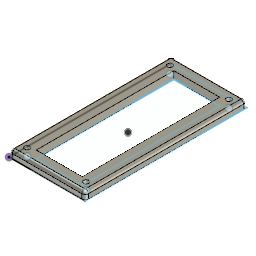
TOP (Autodesk Fusion 360 archive; units mm, degrees)
design "Top lid"
Autodesk Fusion 360 part; units mm, degrees
sketch "Sketch1" plane through (0, 0, 0) normal (0, 0, 1) x (1, 0, 0)
  line L0 (0, 0) -> (40, 0)
  line L1 (40, 0) -> (40, 85)
  line L2 (40, 85) -> (0, 85)
  line L3 (0, 85) -> (0, 0)
  line L4 (7.95, 78.6) -> (32.05, 78.6)
  line L5 (32.05, 78.6) -> (32.05, 6.4)
  line L6 (32.05, 6.4) -> (7.95, 6.4)
  line L7 (7.95, 6.4) -> (7.95, 78.6)
  circle A0 centre (4.5, 80) radius 1.35
  circle A1 centre (4.5, 5) radius 1.35
  circle A2 centre (35.5, 5) radius 1.35
  circle A3 centre (35.5, 80) radius 1.35
  point P0 (20, 42.5)
  point P1 (20, 42.5)
  constraint horizontal L0
  constraint vertical L1
  constraint horizontal L2
  constraint vertical L3
  constraint coincident L0.start L3.end
  constraint horizontal L4
  constraint perpendicular L4 L5
  constraint parallel L4 L6
  constraint parallel L5 L7
  constraint coincident P1 P0
extrude "Extrude1" add sketch "Sketch1" along normal blind 4
fillet "Fillet1" radius 1.5 4 edges at (20, 0, 4) (40, 42.5, 4) (20, 85, 4) (0, 42.5, 4)
fillet "Fillet2" radius 1.75 8 edges at (0, 85, 1.25) (0.4393, 84.5607, 3.5607) (40, 85, 1.25) (39.5607, 84.5607, 3.5607) (39.5607, 0.4393, 3.5607) (40, 0, 1.25) (0.4393, 0.4393, 3.5607) (0, 0, 1.25)
